Autodesk Fusion 360 part; units mm, degrees
note: some values were not read from the file. Set by a fixed rule: which sketch regions a step uses.
(part 5 of 5)
  spline S1306 degree 3 poles (-16.251377, -43.293635) (-16.251377, -42.569588) (-16.843185, -42.084816) (-17.573455, -42.084816) knots 0 0 0 0 1 1 1 1
  line L29 (-17.573455, -42.084816) -> (-20.256193, -42.078282)
  spline S1307 degree 3 poles (-20.256193, -42.078282) (-20.564543, -42.078282) (-20.721985, -41.946043) (-20.721985, -41.675342) knots 0 0 0 0 1 1 1 1
  line L30 (-20.721985, -41.675342) -> (-20.721985, -41.44229)
  spline S1308 degree 3 poles (-20.721985, -41.44229) (-20.721985, -41.215773) (-20.48271, -41.026905) (-20.256193, -41.026905) knots 0 0 0 0 1 1 1 1
  line L31 (-20.256193, -41.026905) -> (-16.23862, -41.026905)
  line L32 (-16.23862, -41.026905) -> (-16.23862, -40.220715)
  line L33 (-16.23862, -40.220715) -> (-20.256193, -40.220715)
  spline S1309 degree 3 poles (-20.256193, -40.220715) (-20.917387, -40.220715) (-21.572047, -40.74967) (-21.572047, -41.44229) knots 0 0 0 0 1 1 1 1
  line L34 (-21.572047, -41.44229) -> (-21.572047, -41.675342)
  spline S1310 degree 3 poles (-21.572047, -41.675342) (-21.572047, -42.386943) (-20.980239, -42.884472) (-20.256193, -42.884472) knots 0 0 0 0 1 1 1 1
  line L35 (-20.256193, -42.884472) -> (-17.573455, -42.890695)
  spline S1311 degree 3 poles (-17.573455, -42.890695) (-17.265105, -42.890695) (-17.107663, -43.022934) (-17.107663, -43.293635) knots 0 0 0 0 1 1 1 1
  line L36 (-17.107663, -43.293635) -> (-17.107663, -43.520463)
  spline S1312 degree 3 poles (-17.107663, -43.520463) (-17.107663, -43.740758) (-17.346938, -43.929626) (-17.573455, -43.929626) knots 0 0 0 0 1 1 1 1
  line L37 (-17.573455, -43.929626) -> (-21.591027, -43.929626)
  line L38 (-21.591027, -43.929626) -> (-21.591027, -44.735505)
  spline S1313 degree 3 poles (-27.83079, -43.513929) (-27.83079, -44.231753) (-27.232759, -44.729282) (-26.514935, -44.729282) knots 0 0 0 0 1 1 1 1
  line L39 (-26.514935, -44.729282) -> (-22.314718, -44.729282)
  line L40 (-22.314718, -44.729282) -> (-22.314718, -40.220714)
  line L41 (-22.314718, -40.220714) -> (-23.165091, -40.220714)
  line L42 (-23.165091, -40.220714) -> (-23.165091, -43.923403)
  line L43 (-23.165091, -43.923403) -> (-26.514935, -43.923403)
  spline S1314 degree 3 poles (-26.514935, -43.923403) (-26.823285, -43.923403) (-26.980727, -43.784941) (-26.980727, -43.513929) knots 0 0 0 0 1 1 1 1
  line L44 (-26.980727, -43.513929) -> (-26.980727, -43.268431)
  spline S1315 degree 3 poles (-26.980727, -43.268431) (-26.980727, -43.016711) (-26.823285, -42.890695) (-26.514935, -42.890695) knots 0 0 0 0 1 1 1 1
  line L45 (-26.514935, -42.890695) -> (-23.429258, -42.890695)
  line L46 (-23.429258, -42.890695) -> (-23.429258, -42.059613)
  line L47 (-23.429258, -42.059613) -> (-26.514935, -42.059613)
  spline S1316 degree 3 poles (-26.514935, -42.059613) (-27.232759, -42.059613) (-27.83079, -42.544385) (-27.83079, -43.268431) knots 0 0 0 0 1 1 1 1
  line L48 (-27.83079, -43.268431) -> (-27.83079, -43.513929)
  spline S1317 degree 3 poles (-34.076987, -43.520463) (-34.076987, -44.194104) (-33.416103, -44.735505) (-32.761132, -44.735505) knots 0 0 0 0 1 1 1 1
  line L49 (-32.761132, -44.735505) -> (-29.914729, -44.735505)
  spline S1318 degree 3 poles (-29.914729, -44.735505) (-29.247312, -44.735505) (-28.592652, -44.194104) (-28.592652, -43.520463) knots 0 0 0 0 1 1 1 1
  line L50 (-28.592652, -43.520463) -> (-28.592652, -41.44229)
  spline S1319 degree 3 poles (-28.592652, -41.44229) (-28.592652, -40.724467) (-29.184459, -40.220714) (-29.914729, -40.220714) knots 0 0 0 0 1 1 1 1
  line L51 (-29.914729, -40.220714) -> (-32.761132, -40.220714)
  spline S1320 degree 3 poles (-32.761132, -40.220714) (-33.472733, -40.220714) (-34.076987, -40.73069) (-34.076987, -41.44229) knots 0 0 0 0 1 1 1 1
  line L52 (-34.076987, -41.44229) -> (-34.076987, -43.520463)
  spline S1321 degree 3 poles (-33.226924, -41.44229) (-33.226924, -41.17159) (-33.069482, -41.039351) (-32.761132, -41.039351) knots 0 0 0 0 1 1 1 1
  line L53 (-32.761132, -41.039351) -> (-29.914729, -41.039351)
  spline S1322 degree 3 poles (-29.914729, -41.039351) (-29.606379, -41.039351) (-29.448937, -41.17159) (-29.448937, -41.44229) knots 0 0 0 0 1 1 1 1
  line L54 (-29.448937, -41.44229) -> (-29.448937, -43.520463)
  spline S1323 degree 3 poles (-29.448937, -43.520463) (-29.448937, -43.740758) (-29.688212, -43.929626) (-29.914729, -43.929626) knots 0 0 0 0 1 1 1 1
  line L55 (-29.914729, -43.929626) -> (-32.761132, -43.929626)
  spline S1324 degree 3 poles (-32.761132, -43.929626) (-32.987649, -43.929626) (-33.226924, -43.740758) (-33.226924, -43.520463) knots 0 0 0 0 1 1 1 1
  line L56 (-33.226924, -43.520463) -> (-33.226924, -41.44229)
  line L57 (-40.140814, -44.735505) -> (-34.88922, -44.735505)
  line L58 (-34.88922, -44.735505) -> (-34.88922, -43.929626)
  line L59 (-34.88922, -43.929626) -> (-37.08034, -43.929626)
  line L60 (-37.08034, -43.929626) -> (-37.08034, -40.220714)
  line L61 (-37.08034, -40.220714) -> (-37.92418, -40.220714)
  line L62 (-37.92418, -40.220714) -> (-37.92418, -43.929626)
  line L63 (-37.92418, -43.929626) -> (-40.140814, -43.929626)
  line L64 (-40.140814, -43.929626) -> (-40.140814, -44.735505)
  line L65 (-46.154039, -44.735505) -> (-40.902444, -44.735505)
  line L66 (-40.902444, -44.735505) -> (-40.902444, -43.929626)
  line L67 (-40.902444, -43.929626) -> (-43.093565, -43.929626)
  line L68 (-43.093565, -43.929626) -> (-43.093565, -40.220714)
  line L69 (-43.093565, -40.220714) -> (-43.937404, -40.220714)
  line L70 (-43.937404, -40.220714) -> (-43.937404, -43.929626)
  line L71 (-43.937404, -43.929626) -> (-46.154039, -43.929626)
  line L72 (-46.154039, -43.929626) -> (-46.154039, -44.735505)
  spline S1325 degree 3 poles (-52.4, -41.688099) (-52.4, -41.977469) (-52.286741, -42.241947) (-52.066447, -42.481221) knots 0 0 0 0 1 1 1 1
  spline S1326 degree 3 poles (-52.066447, -42.481221) (-52.286741, -42.714273) (-52.4, -42.972528) (-52.4, -43.268431) knots 0 0 0 0 1 1 1 1
  line L73 (-52.4, -43.268431) -> (-52.4, -43.513929)
  spline S1327 degree 3 poles (-52.4, -43.513929) (-52.4, -44.231753) (-51.801969, -44.729282) (-51.084145, -44.729282) knots 0 0 0 0 1 1 1 1
  line L74 (-51.084145, -44.729282) -> (-46.883928, -44.729282)
  line L75 (-46.883928, -44.729282) -> (-46.883928, -40.220714)
  line L76 (-46.883928, -40.220714) -> (-47.734301, -40.220714)
  line L77 (-47.734301, -40.220714) -> (-47.734301, -43.923403)
  line L78 (-47.734301, -43.923403) -> (-51.084145, -43.923403)
  spline S1328 degree 3 poles (-51.084145, -43.923403) (-51.392495, -43.923403) (-51.549937, -43.784941) (-51.549937, -43.513929) knots 0 0 0 0 1 1 1 1
  line L79 (-51.549937, -43.513929) -> (-51.549937, -43.268431)
  spline S1329 degree 3 poles (-51.549937, -43.268431) (-51.549937, -43.016711) (-51.392495, -42.890695) (-51.084145, -42.890695) knots 0 0 0 0 1 1 1 1
  line L80 (-51.084145, -42.890695) -> (-47.998468, -42.890695)
  line L81 (-47.998468, -42.890695) -> (-47.998468, -42.059613)
  line L82 (-47.998468, -42.059613) -> (-51.084145, -42.059613)
  spline S1330 degree 3 poles (-51.084145, -42.059613) (-51.329643, -42.059613) (-51.549937, -41.92084) (-51.549937, -41.688099) knots 0 0 0 0 1 1 1 1
  line L83 (-51.549937, -41.688099) -> (-51.549937, -40.220714)
  line L84 (-51.549937, -40.220714) -> (-52.4, -40.220714)
  line L85 (-52.4, -40.220714) -> (-52.4, -41.688099)
extrude "Extrude7" add sketch "LID_LOGO_SPOTTR_SKETCH" along normal blind 0.6 contours S0 S1 S2 S3 S4 S19 S20 S21 S22 S23 S24 S25 S26 S27 S28 S29 S30 S31 S32 S33 S34 S35 S36 S37 S38 S39 S668 S669 S670 S671 S672 S673 S674 S675 S676 S677 S678 S679 S680 S681 S682 S683 S684 S685 S686 S687 S688 S689 S690 S691 S692 S693 S694 S695 S696 S697 S698 S699 S700 | S40 S41 S42 S43 S44 S45 S46 S47 S48 S49 S50 S51 S52 S53 S54 S55 S56 S57 S58 S59 S60 S61 S62 S63 S64 S65 S66 S67 S68 S69 S70 S71 S72 S73 S74 S75 S76 S77 S78 S79 S80 S81 S82 S83 S84 S85 S86 S87 S88 S89 S90 S91 S92 S93 S94 S95 S96 S97 S98 S99 S100 S101 S102 S103 S104 S105 S106 S107 S108 S109 S110 S111 S112 S113 S114 S115 S116 S117 S118 S119 S702 S703 S704 S705 S706 S707 S708 S709 S710 S711 S712 S713 S714 S715 S716 S717 S718 S719 S720 S721 S722 S723 S724 S725 S726 S727 S728 S729 S730 S731 S732 S733 S734 S735 S736 S737 S738 S739 S740 S741 S742 S743 S744 S745 S746 S747 S748 S749 S750 S751 S752 S753 S754 S755 S756 S757 S758 S759 S760 S761 S762 S763 S764 S765 S766 S767 S768 S769 S770 S771 S772 S773 | S120 S121 S122 S123 S124 S125 S126 S127 S128 S129 S130 S131 S132 S133 S134 S135 S136 S137 S138 S139 S140 S141 S142 S143 S144 S145 S146 S147 S148 S149 S150 S151 S152 S153 S154 S155 S156 S157 S158 S159 S160 S161 S162 S163 S164 S165 S166 S167 S168 S169 S170 S171 S172 S173 S174 S175 S176 S177 S178 S179 S180 S181 S182 S183 S184 S185 S186 S187 S188 S189 S190 S191 S192 S193 S194 S195 S196 S197 S198 S199 S200 S201 S202 S203 S204 S205 S206 S207 S208 S209 S210 S211 S212 S213 S214 S215 S216 S782 S783 S784 S785 S786 S787 S788 S789 S790 S791 S792 S793 S794 S795 S796 S797 S798 S799 S800 S801 S802 S803 S804 S805 S806 S807 S808 S809 S810 S811 S812 S813 S814 S815 S816 S817 S818 S819 S820 S821 S822 S823 S824 S825 S838 S839 S840 S841 S842 S843 S844 S845 S846 S847 S848 S849 S850 S851 S852 S853 S854 S855 S856 S857 S858 S859 S860 S861 S862 S863 S864 S865 S866 S867 S868 S869 S870 S871 S872 S873 S874 S875 S876 S877 | S217 S218 S219 S220 S221 S222 S223 S224 S225 S226 S227 S228 S229 S230 S231 S232 S233 S234 S235 S236 S237 S238 S239 S240 S241 S242 S243 S244 S245 S246 S247 S248 S249 S250 S251 S252 S253 L4 S254 S255 S256 S257 S258 S259 S260 S261 L15 S878 S879 S880 S881 S882 S883 S884 S885 S886 S887 S888 S889 S890 S891 S892 S893 S894 S895 S896 S897 S898 S899 S900 S901 S902 S903 S904 S905 S906 S907 S908 S909 S910 S911 S912 S913 S914 S915 S916 S917 S918 S919 S920 S921 S922 | S262 S263 S264 S265 S266 S267 S268 S269 S270 S271 S272 S273 S274 S275 S276 S277 S278 S279 S280 S281 S282 S283 S284 S285 S286 S287 S288 S289 S290 S291 S292 S293 S294 S295 S296 S297 S298 S299 S300 S301 S302 S303 S304 S305 S306 S307 L5 S321 S322 S323 L6 S324 S325 S923 S924 S925 S926 S927 S928 S929 S930 S931 S932 S933 S934 S935 S936 S937 S938 L16 S939 S940 S941 S942 S943 S944 S945 S946 S947 S948 S949 S950 S951 S952 S953 S954 S955 S956 S957 S958 S959 S960 S961 S962 S963 S964 S965 S966 S967 S968 S969 S970 S971 S972 S973 S974 S975 S976 S977 S978 S982 S983 S984 S987 S988 | S322 S323 L6 S324 S325 S985 S986 L17 S987 | S326 L7 S327 S328 S329 S330 S331 S332 S333 S334 S335 S336 S337 S338 S339 S340 S341 S342 S343 S344 L8 S345 L9 S346 S347 S348 S349 S350 S351 S352 S353 S354 S355 S356 S357 L10 S989 S990 S991 S993 L19 S994 S995 S996 S997 S998 S999 S1000 S1001 S1002 S1003 S1004 S1005 S1006 S1007 S1008 S1009 S1010 S1011 L20 S1012 L21 S1013 S1014 S1015 S1016 S1017 S1018 S1019 S1020 | S358 S359 S360 S361 S362 S363 S364 S365 S366 S367 S368 S369 S370 S371 S372 S373 S374 S375 S376 S377 S378 S379 S380 S381 S382 S383 S384 S385 S386 S387 S388 S389 S390 S391 S392 S393 S394 S395 S396 S397 S398 S399 S400 S401 S402 S403 S404 S405 S406 S407 S408 S409 S410 S411 S412 S413 S414 S415 S416 S417 S418 S419 S420 S421 S422 S423 S424 S425 S426 S427 S428 S429 S430 S431 S432 S433 S434 S435 S436 S437 S438 S439 S440 S441 S442 S443 S444 S445 S446 S447 L11 S448 S449 S450 S451 S452 S453 S454 S455 S456 S457 S458 S459 S460 L12 S1021 S1022 S1026 S1027 S1028 S1029 S1030 S1031 S1032 S1033 S1034 S1035 S1036 S1037 S1038 S1039 S1040 S1041 S1042 S1043 S1044 S1045 S1046 S1047 S1048 S1049 S1050 S1051 S1052 S1053 S1054 S1055 S1056 S1057 S1058 S1059 S1060 S1061 S1062 S1063 S1064 S1065 S1066 S1067 S1068 S1069 S1070 S1071 S1072 S1073 S1074 S1075 S1076 S1077 S1078 S1079 S1080 S1081 S1082 S1083 S1084 S1085 S1086 S1087 S1088 S1089 S1090 S1091 S1092 S1093 S1094 S1095 S1096 S1097 S1098 S1099 S1100 S1101 S1102 S1103 S1104 S1105 S1106 S1107 S1108 S1109 S1110 S1111 S1112 S1113 S1114 L24 S1115 S1116 S1117 S1118 S1119 S1120 S1121 S1122 S1123 | S461 S462 S463 S464 S465 S466 S467 S468 S469 S470 S471 S472 S473 S474 S475 S476 S477 S478 S479 S480 S481 S482 S483 S484 S485 S486 S487 S488 S489 S490 S491 S492 S493 S494 S495 S496 S497 S498 S499 S500 S501 S502 S503 S504 S505 S506 S507 S508 S509 S510 S511 S512 S513 S514 S515 S516 S517 S518 S519 S520 S521 S522 S523 S524 S525 S526 S527 S528 S529 S530 S531 S532 S533 S534 S535 S536 S537 S538 S539 S540 S541 S542 S543 S544 S545 S546 S547 S548 S549 S550 S551 S555 S556 S1124 S1128 S1129 S1130 S1131 S1132 S1133 S1134 S1135 S1136 S1137 S1138 S1139 S1140 S1141 S1142 S1143 S1144 S1145 S1146 S1147 S1148 S1149 S1150 S1151 S1152 S1153 S1154 S1155 S1156 S1157 S1158 S1159 S1160 S1161 S1162 S1163 S1164 S1165 S1166 S1167 S1168 S1169 S1170 S1171 S1172 S1173 S1174 S1175 S1176 S1177 S1178 S1179 S1180 S1181 S1182 S1183 S1184 S1185 S1186 S1187 S1188 S1189 S1190 S1191 S1192 S1193 S1194 S1195 S1196 S1197 S1198 S1199 S1200 S1201 S1202 S1203 S1204 S1205 S1206 S1207 S1208 S1209 | S552 S553 S554 S1206 S1207 S1208 | S557 S558 S559 S560 S561 S562 S563 S564 S565 S566 S567 S568 S569 S570 S571 S572 S573 S574 S575 S576 S577 S578 S579 S580 S581 S582 S583 S584 S585 S586 S587 S1210 S1211 S1212 S1213 S1214 S1215 S1216 S1217 S1218 S1219 S1220 S1221 S1222 S1223 S1224 S1225 S1226 S1227 S1228 S1235 S1236 S1237 S1238 S1239 S1240 | S588 S589 S590 S591 S592 S593 S594 S595 S596 S619 S620 S621 S622 S623 S1250 S1251 S1252 S1253 S1254 S1255 S1256 S1257 S1258 S1259 S1260 S1261 S1262 S1263 | S597 S603 S604 S605 S606 S607 S608 S609 S610 S611 S612 S613 S614 S615 S616 S617 S618 S1241 S1242 S1243 S1244 S1245 S1246 S1247 S1248 S1249 S1250 S1251 S1252 S1253 S1254 S1255 S1256 S1257 S1258 S1259 S1260 S1261 S1262 S1263 S1264 S1265 S1266 S1269 S1270 | S614 S615 S1267 S1268 | S629 S630 S631 S632 S633 S634 S635 S636 S637 S638 S639 S640 S641 S642 S643 S644 S645 S646 S647 S648 S649 S650 S651 L13 S652 S653 S654 S655 S656 S657 S658 S659 S660 S1271 S1279 S1280 S1281 S1282 S1283 S1284 L25 S1285 S1286 S1287 S1288 S1289 S1290 S1291 S1292 S1301 S1302 S1303 S1304 | S650 S1301 S1302 | L27 S1305 L28 S1306 L29 S1307 L30 S1308 L31 L32 L33 S1309 L34 S1310 L35 S1311 L36 S1312 L37 L38 | S1313 L39 L40 L41 L42 L43 S1314 L44 S1315 L45 L46 L47 S1316 L48 | S1317 L49 S1318 L50 S1319 L51 S1320 L52 | L57 L58 L59 L60 L61 L62 L63 L64 | L65 L66 L67 L68 L69 L70 L71 L72 | S1325 S1326 L73 S1327 L74 L75 L76 L77 L78 S1328 L79 S1329 L80 L81 L82 S1330 L83 L84 L85 picked at (-9.025166, -50.672157) picked at (-4.096143, -48.114181) picked at (-8.299542, -47.90978) picked at (-2.946894, -44.952032) picked at (-3.582316, -41.755338) picked at (-3.328278, -41.202218) picked at (-11.997701, -39.22895) picked at (-10.451001, -37.413723) picked at (-9.086331, -40.536008) picked at (-5.970227, -35.032701) picked at (-7.763439, -41.83539) picked at (-6.959533, -39.655687) picked at (-4.582735, -35.988229) picked at (-5.824637, -37.361292) picked at (-7.922126, -35.647774) picked at (-8.602626, -36.124667) picked at (-17.577811, -40.758175) picked at (-22.598176, -41.72357) picked at (-30.86353, -40.766472) picked at (-37.651405, -44.466879) picked at (-43.664629, -44.466879) picked at (-47.167385, -42.9578) bodies 1
sketch "USB_CUTOUT_SKETCH" plane through (0, 0, 0) normal (0, -1, 0) x (1, 0, 0)
  line L0 (51, 10.3) -> (3, 10.3)
  line L1 (3, 10.3) -> (3, 0.5)
  line L2 (3, 0.5) -> (51, 0.5)
  line L3 (51, 0.5) -> (51, 10.3)
  line L4 (51, 0.5) -> (3, 0.5)
  line L5 (54, 0.5) -> (54, 10.3) construction
  line L6 (29.825, 7.9) -> (24.325, 7.9)
  arc A0 (24.325, 7.9) -> (24.325, 4) centre (24.325, 5.95) ccw
  line L7 (24.325, 4) -> (29.825, 4)
  arc A1 (29.825, 4) -> (29.825, 7.9) centre (29.825, 5.95) ccw
  line L8 (29.825, 5.95) -> (24.325, 5.95)
  line L9 (51, 11.9) -> (3, 11.9) construction
  line L10 (3, 0) -> (51, 0) construction
  line L11 (3, 11.9) -> (3, 0) construction
  line L12 (3, 5.95) -> (51, 5.95) construction
  point P0 (27, 5.95)
  dimension "d54" = 5.5
  dimension "d55" = 3.9
  constraint tangent L6 A0
  constraint tangent A0 L7
  constraint parallel L6 L7
  constraint tangent L7 A1
  constraint tangent L6 A1
  constraint coincident L9.end L11.start
  constraint coincident L10.start L11.end
  constraint midpoint L11 L12.start
  constraint coincident L3 L12.end
  constraint perpendicular L3 L12
  constraint midpoint L12 P0
  constraint collinear A1.centre A0.centre P0
  measures "d54" distance of A1.centre A0.centre
  measures "d55" distance of L6 L7
extrude "Extrude8" cut sketch "USB_CUTOUT_SKETCH" against normal up to surface (1.6 mm away) contours L6 A0 L7 A1 picked at (27.991667, 5.3) bodies 2
chamfer "Chamfer5" distance 0.3 angle 45 4 edges at (27.075, 0, 7.9) (31.775, 0, 5.95) (27.075, 0, 4) (22.375, 0, 5.95) tangent chain off on bodies 2
equation "CARD_L = 86 mm" comment "Card length"
equation "CARD_W = 54 mm" comment "Card Width"
equation "d3 = CARD_W"
equation "d4 = CARD_L"
equation "BATTERY_T = 9.5 mm" comment "Thickness of Battery"
equation "BATTERY_L = 36 mm" comment "Length of Battery"
equation "BATTERY_W = 26 mm" comment "Width of Battery"
equation "WALL = 1.6 mm" comment "Card Walls"
equation "FLOOR_T = 1.2 mm" comment "Thickness of Card Floor"
equation "LID_T = 1.2 mm" comment "Thickness of Lid"
equation "CARD_T = FLOOR_T + BATTERY_T + LID_T" comment "Total Card Thickness"
equation "d12 = CARD_T"
equation "d15 = CORNER_R"
equation "CORNER_R = 3 mm" comment "Card Corner Radius"
equation "CAVITY_D = BATTERY_T" comment "Depth of the Card Cavity"
equation "d18 = -( FLOOR_T + CAVITY_D )"
equation "d20 = -WALL"
equation "d21 = -CAVITY_D"
equation "LIP_T = 0.8 mm"
equation "LIP_H = 1 mm"
equation "LIP_CLEAR = 0.2 mm"
equation "d26 = -( WALL + LIP_CLEAR )"
equation "d27 = -LIP_T"
equation "d28 = LIP_H"
equation "PCB_Z = 2.2 mm" comment "shim under the board"
equation "PCB_T = 1.25 mm"
equation "USB_H = 3.3 mm"
equation "USB_W = 8.95 mm"
equation "USB_CLEAR = 0.75 mm"
equation "USB_CTR_Z = FLOOR_T + PCB_Z + PCB_T + USB_H / 2"
equation "CHAM_BOT = 0.5 mm"
equation "d55 = USB_H + 0.6 mm"
named bodies: "TOP_LID_BODY", "CARD_BODY"
